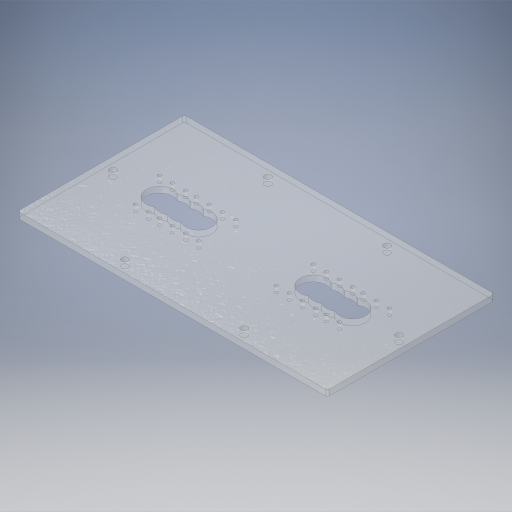
# Autodesk Inventor part: BT001_trajan20_21
Saved by Autodesk Inventor 2023 (Build 270158000, 158)
## iProperties
Company: HTBLA Kaindorf
RuleStatus: InUse
Created: 2022-08-03
Part Number: BT001_trajan20_21
Project: Zeichenmaschine_v2
Material: Acryl
Description: Platte Stepper Motoren
Document SubType Name: Modeling
Designer: trajan20
Density: 1.188 g/cm^3
Appearance: Transparent - farblos
Mass: 201.491 g
Surface Area: 749.507 cm^2
Volume: 169.605 cm^3
AfterDocNew0: iProperties-Editor_aufrufen
Author: jan
Keywords: 2021
Autodesk Inventor part; units mm, degrees
ref_plane "YZ Plane" through (0, 0, 0) normal (1, 0, 0) x (0, 1, 0)
ref_plane "XZ Plane" through (0, 0, 0) normal (0, 1, 0) x (-1, 0, 0)
derived "BT000_trajan20_22_Zeichenmaschine_neu_Masterskizze.ipt"
sketch "Skizze3" plane through (0, 0, 0) normal (0, 0, 1) x (1, 0, 0)
  line L0 (0, 0) -> (-140, 0)
  line L1 (-140, 0) -> (-140, 130)
  line L2 (-140, 260) -> (0, 260)
  line L3 (0, 260) -> (0, 0)
  line L4 (-54.5, 44.5) -> (-85.5, 44.5) construction
  line L5 (-54.5, 75.5) -> (-85.5, 75.5) construction
  line L6 (-85.5, 75.5) -> (-85.5, 44.5) construction
  line L7 (-54.5, 75.5) -> (-54.5, 44.5) construction
  circle A0 centre (-70, 60) radius 11
  circle A1 centre (-85.5, 75.5) radius 1.5
  circle A2 centre (-85.5, 44.5) radius 1.5
  circle A3 centre (-54.5, 44.5) radius 1.5
  circle A4 centre (-54.5, 75.5) radius 1.5
  line L8 (-140, 130) -> (-140, 260)
  circle A5 centre (-70, 71) radius 11
  circle A6 centre (-85.5, 55.5) radius 1.5
  circle A7 centre (-85.5, 86.5) radius 1.5
  circle A8 centre (-85.5, 33.5) radius 1.5
  circle A9 centre (-54.5, 33.5) radius 1.5
  circle A10 centre (-54.5, 55.5) radius 1.5
  circle A11 centre (-85.5, 64.5) radius 1.5
  circle A12 centre (-54.5, 64.5) radius 1.5
  circle A13 centre (-54.5, 86.5) radius 1.5
  circle A14 centre (-70, 49) radius 11
  circle A15 centre (-70, 82) radius 11
  circle A16 centre (-85.5, 97.5) radius 1.5
  circle A17 centre (-54.5, 97.5) radius 1.5
  point P0 (-70, 0)
  point P1 (-70, 10)
  point P2 (-130, 80)
  point P3 (-10, 80)
  point P4 (-60.4737, 65.5)
  point P5 (-79.5263, 65.5)
  point P6 (-79.5263, 54.5)
  point P7 (-60.4737, 54.5)
  point P8 (-60.4737, 76.5)
  point P9 (-79.5263, 76.5)
  dimension "d4" = 260
  dimension "d5" = 140
  dimension "d6" = 31
  dimension "d7" = 31
  dimension "d8" = 15.5
  dimension "d9" = 15.5
  dimension "d10" = 60
  dimension "d11" = 22
  dimension "d12" = 3
  dimension "d13" = 3
  dimension "d14" = 3
  dimension "d15" = 3
  dimension "d22" = 10
  dimension "d23" = 10
  dimension "d26" = 10
  dimension "d57" = 80
  dimension "d61" = 11
  dimension "d62" = 11
  dimension "d63" = 11
  dimension "d64" = 11
  dimension "d65" = 11
  constraints: 26 end point, 16 centre point, 15 vertical alignment, 10 equal radius, 6 horizontal alignment, 5 coincident, 5 point on line, 4 point on circle, 3 horizontal, 3 parallel, 2 perpendicular, 2 vertical, 1 midpoint, 6 other
  measures "d4" distance between parallel lines of L2 L0
  measures "d5" distance between parallel lines of L1 L3
  measures "d6" distance between parallel lines of L6 L7
  measures "d7" distance between parallel lines of L5 L4
  measures "d8" distance from line of L7 point (-70, 60)
  measures "d9" distance from line of L5 point (-70, 60)
  measures "d10" distance from line of L0 point (-70, 60)
  measures "d11" diameter of A0
  measures "d12" diameter of A3
  measures "d13" diameter of A2
  measures "d14" diameter of A4
  measures "d15" diameter of A1
  measures "d22" distance from line of L0 point (-70, 10)
  measures "d23" distance from line of point (-10, 80) L3
  measures "d26" distance from line of L1 point (-130, 80)
  measures "d57" distance from line of L0 point (-130, 80)
  measures "d61" distance of A2.centre A8.centre
  measures "d62" distance of A6.centre A2.centre
  measures "d63" distance of A1.centre A11.centre
  measures "d64" distance of A7.centre A1.centre
  measures "d65" distance of A7.centre A16.centre
extrude "Extrusion3" add sketch "Skizze3" against normal blind 5 contours L0 L1 L8 L2 L3 | A0 A14 A5 | A5 A0 | A0 A15 A5 | A14 A0 | A0 A14 | A0 A5 A15 | A15 A5 | A14 A0 A5 | A15 A5 | A1 | A2 | A3 | A4 | A6 | A7 | A8 | A9 | A10 | A11 | A12 | A13 | A16 | A17
fillet "Rundung1" radius 2 4 edges at (0, 0, -2.5) (0, 260, -2.5) (-140, 260, -2.5) (-140, 0, -2.5)
hole "Bohrung1" at (-70, 10, 0) at (-130, 80, 0) at (-10, 80, 0) direction (0, 0, -1) diameter 5.5 end through all
ref_plane "Arbeitsebene3" through (0, 130, 0) normal (0, 1, 0) x (-1, 0, 0)
extrude "Extrusion6" cut sketch "Skizze3" against normal through all contours A0 A14 A5 | A5 A0 | A0 A15 A5 | A14 A0 | A0 A14 | A0 A5 A15 | A15 A5 | A14 A0 A5 | A15 A5 | A1 | A2 | A3 | A4 | A6 | A7 | A8 | A10 | A11 | A12 | A13 | A16 | A17
mirror "Spiegeln2" about plane through (0, 130, 0) normal (0, 1, 0) of "Extrusion6", "Bohrung1"
equation "\"d8\" = 0.5 * d6"
equation "\"d9\" = d8"
equation "\"d23\" = d22"
equation "\"d26\" = d25"
equation "\"d25\" = d22"
